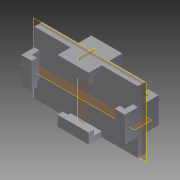
# Autodesk Inventor part: Rover Electronics Raft
Saved by Autodesk Inventor 2012 SP1 (Build 160190100, 190)
## iProperties
Created: 2013-01-31
Part Number: Rover Electronics Raft
Material: Default
Document SubType Name: Modeling
Designer: Administrator
Density: 1 g/cm^3
Author: Administrator
Autodesk Inventor part; units mm, degrees
ref_plane "YZ Plane" through (0, 0, 0) normal (1, 0, 0) x (0, 1, 0)
ref_plane "XZ Plane" through (0, 0, 0) normal (0, 1, 0) x (-1, 0, 0)
ref_plane "XY Plane" through (0, 0, 0) normal (0, 0, 1) x (1, 0, 0)
sketch "Sketch1" plane through (0, 0, 0) normal (0, 0, 1) x (1, 0, 0)
  line L0 (0, 0) -> (127, 0)
  line L1 (127, 0) -> (127, 76.2)
  line L2 (127, 76.2) -> (0, 76.2)
  line L3 (0, 76.2) -> (0, 0)
  dimension "d0" = 127
  dimension "d1" = 76.2
  constraints: 8 end point, 2 parallel, 1 horizontal, 1 perpendicular
  measures "d0" distance of L0.start L0.end
  measures "d1" distance of L2.end L0.start
extrude "Extrusion1" add sketch "Sketch1" along normal blind 9.525
sketch "Sketch2" plane through (0, 0, 9.525) normal (0, 0, 1) x (1, 0, 0)
  line L0 (127, 0) -> (0, 0) projected
  line L1 (0, 76.2) -> (127, 76.2) projected
  line L2 (44.45, 0) -> (82.55, 0)
  line L3 (82.55, 0) -> (82.55, 6.35)
  line L4 (82.55, 6.35) -> (44.45, 6.35)
  line L5 (44.45, 6.35) -> (44.45, 0)
  line L6 (63.5, 76.2) -> (63.5, 0) construction
  dimension "d4" = 38.1
  dimension "d5" = 6.35
  constraints: 10 end point, 2 midpoint, 2 parallel, 2 perpendicular, 1 horizontal, 1 point on line, 1 other
  measures "d4" distance of L3.end L4.end
  measures "d5" distance of L2.end L3.end
extrude "Extrusion2" add sketch "Sketch2" along normal blind 9.525
ref_plane "Work Plane1" through (0, 38.1, 0) normal (0, 1, 0) x (1, 0, 0)
ref_plane "Work Plane2" through (63.5, 0, 0) normal (1, 0, 0) x (0, 0, -1)
sketch "Sketch3" plane through (0, 0, 9.525) normal (0, 0, 1) x (1, 0, 0)
  line L0 (0, 0) -> (0, 76.2) projected
  line L1 (127, 76.2) -> (127, 0) projected
  line L2 (127, 53.975) -> (120.65, 53.975)
  line L3 (120.65, 53.975) -> (120.65, 22.225)
  line L4 (120.65, 22.225) -> (127, 22.225)
  line L5 (127, 22.225) -> (127, 53.975)
  line L6 (0, 38.1) -> (127, 38.1) construction
  point P0 (63.5, 38.1)
  dimension "d8" = 31.75
  dimension "d9" = 6.35
  constraints: 10 end point, 3 midpoint, 2 horizontal, 2 parallel, 2 perpendicular, 1 point on line, 2 other
  measures "d8" distance of L2.end L3.end
  measures "d9" distance of L2.start L2.end
extrude "Extrusion3" add sketch "Sketch3" along normal blind 9.525
sketch "Sketch4" plane through (0, 0, 19.05) normal (0, 0, 1) x (1, 0, 0)
  line L0 (44.45, 0) -> (82.55, 0)
  line L1 (82.55, 0) -> (82.55, 12.7)
  line L2 (82.55, 12.7) -> (44.45, 12.7)
  line L3 (44.45, 12.7) -> (44.45, 0)
  point P0 (44.45, 6.35)
  point P1 (82.55, 6.35)
  point P2 (0, 0)
  dimension "d12" = 38.1
  dimension "d13" = 38.1
  dimension "d14" = 12.7
  constraints: 8 end point, 2 parallel, 1 horizontal, 1 perpendicular
  measures "d12" distance of L1.end L2.end
  measures "d13" distance of point (44.45, 6.35) point (82.55, 6.35)
  measures "d14" distance of L0.end L1.end
extrude "Extrusion4" add sketch "Sketch4" along normal blind 6.35
sketch "Sketch5" plane through (0, 0, 19.05) normal (0, 0, 1) x (1, 0, 0)
  line L0 (127, 53.975) -> (114.3, 53.975)
  line L1 (114.3, 53.975) -> (114.3, 22.225)
  line L2 (114.3, 22.225) -> (127, 22.225)
  line L3 (127, 22.225) -> (127, 53.975)
  point P0 (0, 0)
  dimension "d17" = 31.75
  dimension "d18" = 31.75
  dimension "d19" = 12.7
  constraints: 8 end point, 2 parallel, 1 horizontal, 1 perpendicular
  measures "d17" distance of L0.start point (127, 22.225)
  measures "d18" distance of L0.end L1.end
  measures "d19" distance of L1.end L2.end
extrude "Extrusion5" add sketch "Sketch5" along normal blind 6.35
mirror "Mirror3" about plane through (0, 38.1, 0) normal (0, 1, 0) of "Extrusion2", "Extrusion4"
mirror "Mirror4" about plane through (63.5, 0, 0) normal (1, 0, 0) of "Extrusion3", "Extrusion5"
ref_plane "Work Plane3" through (0, 0, 4.7625) normal (0, 0, 1) x (1, 0, 0)
mirror "Mirror5" about plane through (0, 0, 4.7625) normal (0, 0, 1) of "Extrusion2", "Extrusion4", "Mirror3", "Extrusion3", "Extrusion5", "Mirror4"
equation "\"d12\" = d13"
equation "\"d18\" = d17"
body "Solid1"
